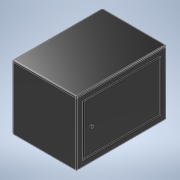
# Autodesk Inventor part: Pieza1
Saved by Autodesk Inventor 2021 (Build 250183000, 183)
## iProperties
Created: 2022-08-16
Part Number: Pieza1
Material: Genérico
Document SubType Name: Modeling
Designer: arthu
Density: 1 g/cm^3
Appearance: Brillante - Negro
Author: arthu
Autodesk Inventor part; units mm, degrees
ref_plane "YZ Plane" through (0, 0, 0) normal (1, 0, 0) x (0, 1, 0)
ref_plane "XZ Plane" through (0, 0, 0) normal (0, 1, 0) x (-1, 0, 0)
ref_plane "XY Plane" through (0, 0, 0) normal (0, 0, 1) x (1, 0, 0)
sketch "Boceto1" plane through (0, 0, 0) normal (0, 0, 1) x (1, 0, 0)
  line L0 (125, 125) -> (-125, 125)
  line L1 (-125, 125) -> (-125, -125)
  line L2 (-125, -125) -> (125, -125)
  line L3 (125, -125) -> (125, 125)
  line L4 (125, 125) -> (-125, -125) construction
  line L5 (-125, 125) -> (125, -125) construction
  point P0 (0, 0)
  dimension "d0" = 250
  dimension "d1" = 250
  constraints: 12 end point, 2 midpoint, 2 parallel, 1 horizontal, 1 perpendicular
  measures "d0" distance of L2.end L1.end
  measures "d1" distance of L1.end L0.end
extrude "Extrusión1" add sketch "Boceto1" along normal blind 350
sketch "Boceto2" plane through (125, -125, 0) normal (1, 0, 0) x (0, 0, -1)
  line L0 (0, 0) -> (0, 250) projected
  line L1 (0, 250) -> (-350, 250) projected
  line L2 (-350, 0) -> (-350, 250) projected
  line L3 (0, 0) -> (-350, 0) projected
  line L4 (-325, 225) -> (-25, 225)
  line L5 (-25, 225) -> (-25, 25)
  line L6 (-25, 25) -> (-325, 25)
  line L7 (-325, 25) -> (-325, 225)
  line L8 (-30, 220) -> (-320, 220)
  line L9 (-320, 220) -> (-320, 30)
  line L10 (-320, 30) -> (-30, 30)
  line L11 (-30, 30) -> (-30, 220)
  point P0 (0, 125)
  dimension "d4" = 25
  dimension "d5" = 5
  constraints: 16 end point, 6 other
  measures "d4" distance between parallel lines of L1 L4
  measures "d5" distance between parallel lines of L4 L8
extrude "Extrusión2" cut sketch "Boceto2" against normal blind 5 contours L4 L5 L6 L7
sketch "Boceto3" plane through (125, -95, 30) normal (1, 0, 0) x (0, 0, -1)
  line L0 (-290, 0) -> (0, 0) projected
  line L1 (0, 0) -> (0, 190) projected
  line L2 (0, 190) -> (-290, 190) projected
  line L3 (-290, 190) -> (-290, 0) projected
  circle A0 centre (-263.8975, 95) radius 5
  point P0 (30, 95)
  dimension "d8" = 10
  constraints: 1 centre point
  measures "d8" diameter of A0
extrude "Extrusión3" add sketch "Boceto3" along normal blind 5 contours A0
fillet "Empalme1" radius 5 12 edges at (0, 125, 350) (0, 125, 0) (0, -125, 350) (0, -125, 0) (-125, 125, 175) (-125, 0, 0) (-125, 0, 350) (-125, -125, 175) (125, 0, 350) (125, 125, 175) (125, 0, 0) (125, -125, 175)
